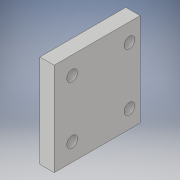
# Autodesk Inventor part: cLIMPpLATE
Saved by Autodesk Inventor 2019 (Build 230136000, 136)
## iProperties
Created: 2019-10-03
Part Number: cLIMPpLATE
Material: Generic
Document SubType Name: Modeling
Designer: james
Density: 1 g/cm^3
Appearance: Default
Author: james
Autodesk Inventor part; units mm, degrees
ref_plane "YZ Plane" through (0, 0, 0) normal (1, 0, 0) x (0, 1, 0)
ref_plane "XZ Plane" through (0, 0, 0) normal (0, 1, 0) x (-1, 0, 0)
ref_plane "XY Plane" through (0, 0, 0) normal (0, 0, 1) x (1, 0, 0)
sketch "Sketch1" plane through (0, 0, 0) normal (1, 0, 0) x (0, 1, 0)
  line L0 (-12.564, -8.5827) -> (20.456, -8.5827)
  line L1 (20.456, -8.5827) -> (20.456, 21.8973)
  line L2 (20.456, 21.8973) -> (-12.564, 21.8973)
  line L3 (-12.564, 21.8973) -> (-12.564, -8.5827)
  point P0 (0, 0)
  dimension "d0" = 30.48
  dimension "d1" = 33.02
  constraints: 8 end point, 2 parallel, 1 horizontal, 1 perpendicular
  measures "d0" distance of L2.end L0.start
  measures "d1" distance of L1.end L2.end
extrude "Extrusion1" add sketch "Sketch1" along normal blind 5.08
sketch "Sketch2" plane through (5.08, 0, 0) normal (1, 0, 0) x (0, 0, -1)
  line L0 (8.5827, -12.564) -> (8.5827, 20.456) projected
  line L1 (-21.8973, -12.564) -> (8.5827, -12.564) projected
  line L2 (8.5827, 20.456) -> (-21.8973, 20.456) projected
  line L3 (-21.8973, 20.456) -> (-21.8973, -12.564) projected
  point P0 (0, 0)
  point P1 (4.7727, 14.106)
  point P2 (-15.5473, 14.106)
  point P3 (-15.5473, -6.214)
  point P4 (4.7727, -6.214)
  dimension "d4" = 3.81
  dimension "d5" = 3.81
  dimension "d6" = 6.35
  dimension "d7" = 6.35
  dimension "d8" = 6.35
  dimension "d9" = 6.35
  dimension "d10" = 6.35
  dimension "d11" = 6.35
  measures "d4" distance from line of L0 point (4.773, 14.106)
  measures "d5" distance from line of L0 point (4.773, -6.214)
  measures "d6" distance from line of L1 point (4.773, -6.214)
  measures "d7" distance from line of L2 point (4.773, 14.106)
  measures "d8" distance from line of L3 point (-15.547, 14.106)
  measures "d9" distance from line of L2 point (-15.547, 14.106)
  measures "d10" distance from line of L1 point (-15.547, -6.214)
  measures "d11" distance from line of point (-15.547, -6.214) L3
hole "Hole1" at (5.08, 14.106, -4.7727) at (5.08, 14.106, 15.5473) at (5.08, -6.214, 15.5473) at (5.08, -6.214, -4.7727) direction (-1, 0, 0) diameter 3.81 depth 10.9728 tip angle 118.188 clearance for "Flat Head Machine Screw (82)" size "#6" standard "Ansi Unified Screw Threads"
body "Solid1"
